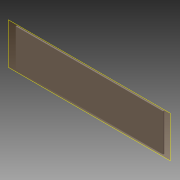
# Autodesk Inventor part: Panel_back
Saved by Autodesk Inventor 2013 (Build 170138000, 138)
## iProperties
Created: 2013-01-31
Part Number: Panel_back
Material: Generic
Document SubType Name: Modeling
Designer: xylzlyx
Density: 1 g/cm^3
Author: xylzlyx
Autodesk Inventor part; units mm, degrees
ref_plane "YZ Plane" through (0, 0, 0) normal (1, 0, 0) x (0, 1, 0)
ref_plane "XZ Plane" through (0, 0, 0) normal (0, 1, 0) x (-1, 0, 0)
ref_plane "XY Plane" through (0, 0, 0) normal (0, 0, 1) x (1, 0, 0)
ref_plane "Work Plane1" through (0, 0, 0) normal (0, 0, 1) x (1, 0, 0)
sketch "Sketch3" plane through (0, 0, 0) normal (0, 0, 1) x (1, 0, 0)
  line L0 (-3, 1.9994) -> (-3, 94.9117) construction
  line L1 (-2, 0) -> (-373, 0) construction
  line L2 (-2, 97.6432) -> (-373, 97.6432) construction
  line L3 (-372, 94.9117) -> (-372, 1.9994) construction
  line L4 (-372, 93.6432) -> (-3, 93.6432)
  line L5 (-3, 93.6432) -> (-3, 0)
  line L6 (-3, 0) -> (-372, 0)
  line L7 (-372, 0) -> (-372, 93.6432)
  point P0 (0, 0)
  point P1 (-187.5, 0)
  point P2 (-3, 48.4555)
  point P3 (-372, 0)
  point P4 (-372, 48.4555)
  dimension "d3" = 4
  constraints: 8 end point, 4 point on line, 4 vertical alignment, 3 midpoint, 2 horizontal alignment, 2 parallel, 1 horizontal, 1 perpendicular
  measures "d3" distance between parallel lines of L2 L4
extrude "Extrusion1" add sketch "Sketch3" against normal blind 3
body "Solid1"
